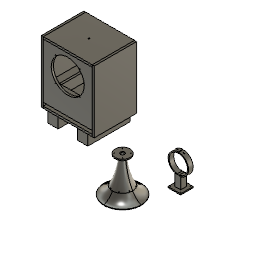
speaker-full-design (Autodesk Fusion 360 design; units mm, degrees)
Autodesk Fusion 360 part; units mm, degrees
sketch "HornProfile" plane through (0, 0, 0) normal (0, 1, 0) x (1, 0, 0)
  spline S0 degree 5 poles (18, 0) (18.0182, 0.1631) (18.0556, 0.496) (18.1141, 1.0154) (18.1973, 1.7477) (18.3097, 2.7291) (18.4304, 3.7743) (18.5588, 4.8793) (18.6943, 6.0374) (18.8359, 7.2396) (18.9826, 8.4763) (19.1333, 9.7379) (19.2872, 11.0163) (19.4438, 12.3059) (19.6027, 13.6042) (19.764, 14.9104) (19.9278, 16.2251) (20.0942, 17.5496) (20.2635, 18.8851) (20.4356, 20.2317) (20.6106, 21.5889) (20.7883, 22.9555) (20.9685, 24.3298) (21.1511, 25.7103) (21.3359, 27.0955) (21.5229, 28.4844) (21.7119, 29.8765) (21.903, 31.2715) (22.0963, 32.6694) (22.2917, 34.0701) (22.4893, 35.4739) (22.6891, 36.8805) (22.8911, 38.2897) (23.0954, 39.7013) (23.3018, 41.1147) (23.5104, 42.5296) (23.721, 43.9456) (23.9337, 45.3623) (24.1485, 46.7795) (24.3653, 48.1969) (24.5841, 49.6145) (24.8048, 51.0322) (25.0276, 52.4497) (25.2523, 53.8671) (25.4789, 55.2843) (25.7076, 56.701) (25.9382, 58.1171) (26.1709, 59.5326) (26.4056, 60.9472) (26.6423, 62.3607) (26.881, 63.7732) (27.1218, 65.1844) (27.3646, 66.5942) (27.6094, 68.0027) (27.8562, 69.4096) (28.1051, 70.8149) (28.3559, 72.2186) (28.6086, 73.6205) (28.8634, 75.0205) (29.12, 76.4187) (29.3787, 77.8149) (29.6393, 79.209) (29.9019, 80.6009) (30.1664, 81.9907) (30.4329, 83.3782) (30.7015, 84.7635) (30.972, 86.1463) (31.2446, 87.5268) (31.5193, 88.9048) (31.796, 90.2803) (32.0747, 91.6533) (32.3554, 93.0236) (32.6382, 94.3914) (32.923, 95.7564) (33.2098, 97.1188) (33.4986, 98.4784) (33.7894, 99.8352) (34.0822, 101.1892) (34.377, 102.5404) (34.6739, 103.8886) (34.9728, 105.234) (35.2737, 106.5763) (35.5767, 107.9157) (35.8817, 109.2521) (36.1887, 110.5855) (36.4978, 111.9158) (36.8089, 113.2431) (37.1221, 114.5672) (37.4374, 115.8882) (37.7548, 117.206) (38.0742, 118.5207) (38.3958, 119.8321) (38.7195, 121.1402) (39.0453, 122.4451) (39.3731, 123.7468) (39.703, 125.0451) (40.035, 126.3402) (40.3691, 127.6319) (40.7052, 128.9203) (41.0434, 130.2054) (41.3837, 131.4872) (41.7261, 132.7655) (42.0706, 134.0405) (42.4173, 135.312) (42.7661, 136.5802) (43.1172, 137.8448) (43.4704, 139.1061) (43.8258, 140.3639) (44.1834, 141.6182) (44.5432, 142.8691) (44.9051, 144.1166) (45.2692, 145.3605) (45.6354, 146.601) (46.0038, 147.8379) (46.3742, 149.0713) (46.7469, 150.3012) (47.1216, 151.5274) (47.4986, 152.7501) (47.8777, 153.9692) (48.259, 155.1847) (48.6425, 156.3966) (49.0283, 157.6049) (49.4163, 158.8096) (49.8065, 160.0107) (50.199, 161.2082) (50.5937, 162.4021) (50.9907, 163.5923) (51.3899, 164.779) (51.7913, 165.962) (52.195, 167.1413) (52.601, 168.317) (53.0092, 169.489) (53.4196, 170.6573) (53.8323, 171.8219) (54.2472, 172.9828) (54.6644, 174.14) (55.0838, 175.2935) (55.5055, 176.4433) (55.9295, 177.5894) (56.3557, 178.7317) (56.7843, 179.8702) (57.2153, 181.005) (57.6485, 182.136) (58.0842, 183.2632) (58.5222, 184.3866) (58.9625, 185.5062) (59.4051, 186.6222) (59.85, 187.7344) (60.2973, 188.8429) (60.7468, 189.9476) (61.1986, 191.0485) (61.6528, 192.1456) (62.1093, 193.2387) (62.5682, 194.328) (63.0294, 195.4134) (63.493, 196.4949) (63.959, 197.5725) (64.4274, 198.6463) (64.8982, 199.7163) (65.3713, 200.7825) (65.8469, 201.8448) (66.3248, 202.9033) (66.8051, 203.9579) (67.2879, 205.0085) (67.7731, 206.0552) (68.2607, 207.098) (68.7508, 208.1367) (69.2432, 209.1715) (69.7381, 210.2022) (70.2355, 211.229) (70.7353, 212.2518) (71.2375, 213.2707) (71.7422, 214.2855) (72.2493, 215.2964) (72.7589, 216.3032) (73.2711, 217.3061) (73.7857, 218.3049) (74.3028, 219.2997) (74.8225, 220.2904) (75.3446, 221.2771) (75.8692, 222.2597) (76.3962, 223.2382) (76.9256, 224.2126) (77.4575, 225.1829) (77.9918, 226.1491) (78.5286, 227.1111) (79.068, 228.0689) (79.6101, 229.0226) (80.1547, 229.9721) (80.702, 230.9174) (81.2518, 231.8585) (81.8041, 232.7954) (82.3589, 233.7281) (82.9162, 234.6566) (83.4759, 235.5808) (84.0382, 236.5007) (84.6031, 237.4163) (85.1705, 238.3276) (85.7407, 239.2346) (86.3134, 240.1371) (86.8888, 241.0353) (87.4668, 241.9291) (88.0473, 242.8185) (88.6305, 243.7035) (89.2162, 244.584) (89.8046, 245.46) (90.3956, 246.3316) (90.9893, 247.1987) (91.5856, 248.0613) (92.1845, 248.9195) (92.7861, 249.7731) (93.3903, 250.6223) (93.9971, 251.4669) (94.6066, 252.3068) (95.2187, 253.1421) (95.8334, 253.9726) (96.4508, 254.7984) (97.0709, 255.6194) (97.6936, 256.4356) (98.3191, 257.2471) (98.9473, 258.0539) (99.5782, 258.856) (100.2118, 259.6533) (100.8481, 260.4457) (101.4872, 261.2331) (102.1289, 262.0156) (102.7733, 262.7931) (103.4203, 263.5655) (104.07, 264.333) (104.7224, 265.0955) (105.3775, 265.853) (106.0354, 266.6053) (106.6961, 267.3526) (107.3596, 268.0946) (108.0259, 268.8313) (108.6951, 269.5628) (109.367, 270.289) (110.0416, 271.0098) (110.7189, 271.7253) (111.3989, 272.4355) (112.0817, 273.1401) (112.7674, 273.8392) (113.4559, 274.5328) (114.1473, 275.2207) (114.8415, 275.903) (115.5385, 276.5797) (116.2382, 277.2507) (116.9406, 277.916) (117.6458, 278.5755) (118.3539, 279.2291) (119.0648, 279.8767) (119.7786, 280.5183) (120.4953, 281.1537) (121.2148, 281.783) (121.9372, 282.4062) (122.6623, 283.0231) (123.3903, 283.6337) (124.1212, 284.2379) (124.855, 284.8357) (125.5918, 285.4269) (126.3316, 286.0114) (127.0742, 286.5893) (127.8197, 287.1603) (128.5679, 287.7245) (129.3189, 288.2817) (130.0727, 288.8319) (130.8295, 289.3751) (131.5893, 289.9111) (132.3522, 290.4399) (133.118, 290.9611) (133.8868, 291.4747) (134.6585, 291.9805) (135.4331, 292.4784) (136.2105, 292.9683) (136.9908, 293.4501) (137.7741, 293.9238) (138.5603, 294.3893) (139.3495, 294.8464) (140.1417, 295.2948) (140.9369, 295.7343) (141.7351, 296.1647) (142.5363, 296.5857) (143.3405, 296.9972) (144.1476, 297.3988) (144.9577, 297.7905) (145.7708, 298.1719) (146.587, 298.5428) (147.4062, 298.9029) (148.2284, 299.2517) (149.0536, 299.5887) (149.8818, 299.9134) (150.7129, 300.2253) (151.547, 300.5242) (152.3841, 300.8099) (153.2243, 301.082) (154.0677, 301.3397) (154.9142, 301.5811) (155.7639, 301.8038) (156.6167, 302.0054) (157.4725, 302.1836) (158.3314, 302.337) (159.0209, 302.4394) (159.5394, 302.5047) (159.8857, 302.5431) (160.059, 302.561) knots 0 0 0 0 0 0 0.00333333 0.00666667 0.01 0.01333333 0.01666667 0.02 0.02333333 0.02666667 0.03 0.03333333 0.03666667 0.04 0.04333333 0.04666667 0.05 0.05333333 0.05666667 0.06 0.06333333 0.06666667 0.07 0.07333333 0.07666667 0.08 0.08333333 0.08666667 0.09 0.09333333 0.09666667 0.1 0.10333333 0.10666667 0.11 0.11333333 0.11666667 0.12 0.12333333 0.12666667 0.13 0.13333333 0.13666667 0.14 0.14333333 0.14666667 0.15 0.15333333 0.15666667 0.16 0.16333333 0.16666667 0.17 0.17333333 0.17666667 0.18 0.18333333 0.18666667 0.19 0.19333333 0.19666667 0.2 0.20333333 0.20666667 0.21 0.21333333 0.21666667 0.22 0.22333333 0.22666667 0.23 0.23333333 0.23666667 0.24 0.24333333 0.24666667 0.25 0.25333333 0.25666667 0.26 0.26333333 0.26666667 0.27 0.27333333 0.27666667 0.28 0.28333333 0.28666667 0.29 0.29333333 0.29666667 0.3 0.30333333 0.30666667 0.31 0.31333333 0.31666667 0.32 0.32333333 0.32666667 0.33 0.33333333 0.33666667 0.34 0.34333333 0.34666667 0.35 0.35333333 0.35666667 0.36 0.36333333 0.36666667 0.37 0.37333333 0.37666667 0.38 0.38333333 0.38666667 0.39 0.39333333 0.39666667 0.4 0.40333333 0.40666667 0.41 0.41333333 0.41666667 0.42 0.42333333 0.42666667 0.43 0.43333333 0.43666667 0.44 0.44333333 0.44666667 0.45 0.45333333 0.45666667 0.46 0.46333333 0.46666667 0.47 0.47333333 0.47666667 0.48 0.48333333 0.48666667 0.49 0.49333333 0.49666667 0.5 0.50333333 0.50666667 0.51 0.51333333 0.51666667 0.52 0.52333333 0.52666667 0.53 0.53333333 0.53666667 0.54 0.54333333 0.54666667 0.55 0.55333333 0.55666667 0.56 0.56333333 0.56666667 0.57 0.57333333 0.57666667 0.58 0.58333333 0.58666667 0.59 0.59333333 0.59666667 0.6 0.60333333 0.60666667 0.61 0.61333333 0.61666667 0.62 0.62333333 0.62666667 0.63 0.63333333 0.63666667 0.64 0.64333333 0.64666667 0.65 0.65333333 0.65666667 0.66 0.66333333 0.66666667 0.67 0.67333333 0.67666667 0.68 0.68333333 0.68666667 0.69 0.69333333 0.69666667 0.7 0.70333333 0.70666667 0.71 0.71333333 0.71666667 0.72 0.72333333 0.72666667 0.73 0.73333333 0.73666667 0.74 0.74333333 0.74666667 0.75 0.75333333 0.75666667 0.76 0.76333333 0.76666667 0.77 0.77333333 0.77666667 0.78 0.78333333 0.78666667 0.79 0.79333333 0.79666667 0.8 0.80333333 0.80666667 0.81 0.81333333 0.81666667 0.82 0.82333333 0.82666667 0.83 0.83333333 0.83666667 0.84 0.84333333 0.84666667 0.85 0.85333333 0.85666667 0.86 0.86333333 0.86666667 0.87 0.87333333 0.87666667 0.88 0.88333333 0.88666667 0.89 0.89333333 0.89666667 0.9 0.90333333 0.90666667 0.91 0.91333333 0.91666667 0.92 0.92333333 0.92666667 0.93 0.93333333 0.93666667 0.94 0.94333333 0.94666667 0.95 0.95333333 0.95666667 0.96 0.96333333 0.96666667 0.97 0.97333333 0.97666667 0.98 0.98333333 0.98666667 0.99 0.99333333 0.99666667 1 1 1 1 1 1
  spline S1 degree 5 poles (23.961, -0.681) (23.9791, -0.5202) (24.016, -0.1922) (24.0738, 0.3193) (24.1559, 1.0402) (24.2665, 2.0055) (24.3851, 3.033) (24.5111, 4.1191) (24.6441, 5.2572) (24.783, 6.4388) (24.9269, 7.6547) (25.0748, 8.8956) (25.2261, 10.1535) (25.3799, 11.4227) (25.5362, 12.7005) (25.6948, 13.986) (25.8559, 15.2796) (26.0194, 16.5826) (26.1857, 17.8961) (26.3548, 19.2205) (26.5266, 20.5553) (26.7011, 21.8994) (26.878, 23.2514) (27.0574, 24.6097) (27.239, 25.9729) (27.4227, 27.3398) (27.6085, 28.7098) (27.7963, 30.0826) (27.9862, 31.4583) (28.1782, 32.8367) (28.3723, 34.218) (28.5685, 35.6021) (28.7669, 36.9889) (28.9672, 38.378) (29.1697, 39.7691) (29.3742, 41.1617) (29.5807, 42.5554) (29.7891, 43.9499) (29.9996, 45.3448) (30.212, 46.74) (30.4263, 48.1354) (30.6427, 49.5309) (30.861, 50.9263) (31.0814, 52.3215) (31.3037, 53.7166) (31.528, 55.1113) (31.7542, 56.5054) (31.9825, 57.8989) (32.2126, 59.2915) (32.4448, 60.6832) (32.6788, 62.0737) (32.9148, 63.463) (33.1527, 64.851) (33.3925, 66.2376) (33.6342, 67.6228) (33.8778, 69.0064) (34.1234, 70.3884) (34.3708, 71.7688) (34.6203, 73.1473) (34.8717, 74.524) (35.125, 75.8987) (35.3803, 77.2714) (35.6376, 78.642) (35.8969, 80.0104) (36.158, 81.3766) (36.4211, 82.7406) (36.6861, 84.1022) (36.953, 85.4615) (37.2218, 86.8185) (37.4925, 88.173) (37.7651, 89.5251) (38.0396, 90.8746) (38.316, 92.2216) (38.5945, 93.566) (38.8749, 94.9077) (39.1574, 96.2466) (39.4419, 97.5828) (39.7284, 98.9162) (40.0169, 100.2467) (40.3074, 101.5744) (40.5998, 102.8991) (40.8942, 104.221) (41.1906, 105.5399) (41.4889, 106.8558) (41.7892, 108.1688) (42.0914, 109.4788) (42.3957, 110.7858) (42.7019, 112.0897) (43.0101, 113.3906) (43.3203, 114.6884) (43.6325, 115.9831) (43.9466, 117.2746) (44.2627, 118.5628) (44.5808, 119.8479) (44.9008, 121.1297) (45.223, 122.4083) (45.5472, 123.6836) (45.8735, 124.9557) (46.202, 126.2245) (46.5325, 127.49) (46.8652, 128.7522) (47.1999, 130.0111) (47.5366, 131.2666) (47.8754, 132.5188) (48.2161, 133.7676) (48.5588, 135.0129) (48.9035, 136.2548) (49.2502, 137.4933) (49.599, 138.7284) (49.9499, 139.9601) (50.3029, 141.1883) (50.6581, 142.4131) (51.0155, 143.6344) (51.375, 144.8522) (51.7365, 146.0666) (52.1002, 147.2775) (52.4659, 148.4848) (52.8337, 149.6887) (53.2036, 150.8889) (53.5756, 152.0857) (53.9497, 153.2789) (54.326, 154.4685) (54.7044, 155.6545) (55.0849, 156.837) (55.4676, 158.016) (55.8524, 159.1913) (56.2394, 160.3631) (56.6284, 161.5313) (57.0195, 162.6959) (57.4128, 163.8569) (57.8082, 165.0143) (58.2058, 166.168) (58.6057, 167.318) (59.0077, 168.4644) (59.4119, 169.607) (59.8184, 170.746) (60.2271, 171.8813) (60.638, 173.0129) (61.0511, 174.1409) (61.4664, 175.2651) (61.8839, 176.3857) (62.3037, 177.5025) (62.7257, 178.6156) (63.15, 179.725) (63.5765, 180.8307) (64.0052, 181.9326) (64.4361, 183.0307) (64.8691, 184.1252) (65.3043, 185.2158) (65.7416, 186.3028) (66.1811, 187.3859) (66.623, 188.4653) (67.0671, 189.5408) (67.5136, 190.6125) (67.9625, 191.6804) (68.4137, 192.7444) (68.8673, 193.8046) (69.3232, 194.8609) (69.7813, 195.9135) (70.2416, 196.9622) (70.7041, 198.0071) (71.1687, 199.0483) (71.6357, 200.0855) (72.1049, 201.1189) (72.5765, 202.1484) (73.0504, 203.174) (73.5268, 204.1957) (74.0055, 205.2134) (74.4866, 206.2271) (74.97, 207.2369) (75.4558, 208.2427) (75.9439, 209.2446) (76.4344, 210.2425) (76.9271, 211.2364) (77.4222, 212.2264) (77.9196, 213.2125) (78.4192, 214.1945) (78.9212, 215.1727) (79.4256, 216.1468) (79.9323, 217.1168) (80.4414, 218.0828) (80.9529, 219.0447) (81.4668, 220.0025) (81.9832, 220.9561) (82.502, 221.9056) (83.0233, 222.851) (83.547, 223.7923) (84.0731, 224.7295) (84.6015, 225.6626) (85.1322, 226.5916) (85.6653, 227.5164) (86.2008, 228.4371) (86.7388, 229.3535) (87.2793, 230.2657) (87.8223, 231.1736) (88.3678, 232.0772) (88.9159, 232.9764) (89.4663, 233.8714) (90.0192, 234.7622) (90.5744, 235.6487) (91.132, 236.531) (91.6919, 237.409) (92.2542, 238.2826) (92.8189, 239.1518) (93.3861, 240.0167) (93.9559, 240.877) (94.5282, 241.7329) (95.103, 242.5843) (95.6805, 243.4311) (96.2605, 244.2735) (96.843, 245.1113) (97.428, 245.9447) (98.0153, 246.7735) (98.605, 247.5979) (99.1972, 248.4177) (99.7918, 249.2329) (100.389, 250.0434) (100.9888, 250.8493) (101.5912, 251.6503) (102.1961, 252.4467) (102.8036, 253.2382) (103.4135, 254.0248) (104.026, 254.8067) (104.6409, 255.5837) (105.2584, 256.3559) (105.8783, 257.1233) (106.5008, 257.8859) (107.1258, 258.6435) (107.7534, 259.3962) (108.3835, 260.144) (109.0162, 260.8866) (109.6513, 261.6241) (110.2891, 262.3565) (110.9294, 263.0838) (111.5723, 263.8058) (112.2178, 264.5226) (112.8659, 265.2341) (113.5166, 265.9404) (114.1698, 266.6414) (114.8255, 267.337) (115.4838, 268.0272) (116.1446, 268.712) (116.8079, 269.3912) (117.4739, 270.0649) (118.1425, 270.7329) (118.8137, 271.3953) (119.4874, 272.0521) (120.1636, 272.7032) (120.8424, 273.3486) (121.5236, 273.9882) (122.2074, 274.6218) (122.8938, 275.2495) (123.5828, 275.8711) (124.2744, 276.4866) (124.9686, 277.096) (125.6653, 277.6991) (126.3646, 278.296) (127.0664, 278.8866) (127.7707, 279.4707) (128.4775, 280.0484) (129.1869, 280.6195) (129.8989, 281.1839) (130.6134, 281.7416) (131.3304, 282.2925) (132.0499, 282.8366) (132.772, 283.3738) (133.4966, 283.9039) (134.2238, 284.4267) (134.9534, 284.942) (135.6856, 285.4499) (136.4202, 285.9502) (137.1571, 286.443) (137.8963, 286.9282) (138.6378, 287.4057) (139.3817, 287.8752) (140.1281, 288.3365) (140.877, 288.7894) (141.6283, 289.2336) (142.3818, 289.6691) (143.1375, 290.0958) (143.8951, 290.5134) (144.6548, 290.9219) (145.4168, 291.3209) (146.1812, 291.7101) (146.948, 292.0892) (147.7168, 292.458) (148.487, 292.8162) (149.2581, 293.1636) (150.03, 293.4998) (150.8036, 293.8244) (151.5798, 294.1369) (152.3591, 294.4366) (153.1407, 294.723) (153.9218, 294.9956) (154.6993, 295.2535) (155.4713, 295.4961) (156.2386, 295.722) (157.0056, 295.9295) (157.778, 296.1169) (158.5615, 296.2827) (159.36, 296.4258) (160.0121, 296.5219) (160.509, 296.5835) (160.8438, 296.62) (161.012, 296.637) knots 0 0 0 0 0 0 0.00333333 0.00666667 0.01 0.01333333 0.01666667 0.02 0.02333333 0.02666667 0.03 0.03333333 0.03666667 0.04 0.04333333 0.04666667 0.05 0.05333333 0.05666667 0.06 0.06333333 0.06666667 0.07 0.07333333 0.07666667 0.08 0.08333333 0.08666667 0.09 0.09333333 0.09666667 0.1 0.10333333 0.10666667 0.11 0.11333333 0.11666667 0.12 0.12333333 0.12666667 0.13 0.13333333 0.13666667 0.14 0.14333333 0.14666667 0.15 0.15333333 0.15666667 0.16 0.16333333 0.16666667 0.17 0.17333333 0.17666667 0.18 0.18333333 0.18666667 0.19 0.19333333 0.19666667 0.2 0.20333333 0.20666667 0.21 0.21333333 0.21666667 0.22 0.22333333 0.22666667 0.23 0.23333333 0.23666667 0.24 0.24333333 0.24666667 0.25 0.25333333 0.25666667 0.26 0.26333333 0.26666667 0.27 0.27333333 0.27666667 0.28 0.28333333 0.28666667 0.29 0.29333333 0.29666667 0.3 0.30333333 0.30666667 0.31 0.31333333 0.31666667 0.32 0.32333333 0.32666667 0.33 0.33333333 0.33666667 0.34 0.34333333 0.34666667 0.35 0.35333333 0.35666667 0.36 0.36333333 0.36666667 0.37 0.37333333 0.37666667 0.38 0.38333333 0.38666667 0.39 0.39333333 0.39666667 0.4 0.40333333 0.40666667 0.41 0.41333333 0.41666667 0.42 0.42333333 0.42666667 0.43 0.43333333 0.43666667 0.44 0.44333333 0.44666667 0.45 0.45333333 0.45666667 0.46 0.46333333 0.46666667 0.47 0.47333333 0.47666667 0.48 0.48333333 0.48666667 0.49 0.49333333 0.49666667 0.5 0.50333333 0.50666667 0.51 0.51333333 0.51666667 0.52 0.52333333 0.52666667 0.53 0.53333333 0.53666667 0.54 0.54333333 0.54666667 0.55 0.55333333 0.55666667 0.56 0.56333333 0.56666667 0.57 0.57333333 0.57666667 0.58 0.58333333 0.58666667 0.59 0.59333333 0.59666667 0.6 0.60333333 0.60666667 0.61 0.61333333 0.61666667 0.62 0.62333333 0.62666667 0.63 0.63333333 0.63666667 0.64 0.64333333 0.64666667 0.65 0.65333333 0.65666667 0.66 0.66333333 0.66666667 0.67 0.67333333 0.67666667 0.68 0.68333333 0.68666667 0.69 0.69333333 0.69666667 0.7 0.70333333 0.70666667 0.71 0.71333333 0.71666667 0.72 0.72333333 0.72666667 0.73 0.73333333 0.73666667 0.74 0.74333333 0.74666667 0.75 0.75333333 0.75666667 0.76 0.76333333 0.76666667 0.77 0.77333333 0.77666667 0.78 0.78333333 0.78666667 0.79 0.79333333 0.79666667 0.8 0.80333333 0.80666667 0.81 0.81333333 0.81666667 0.82 0.82333333 0.82666667 0.83 0.83333333 0.83666667 0.84 0.84333333 0.84666667 0.85 0.85333333 0.85666667 0.86 0.86333333 0.86666667 0.87 0.87333333 0.87666667 0.88 0.88333333 0.88666667 0.89 0.89333333 0.89666667 0.9 0.90333333 0.90666667 0.91 0.91333333 0.91666667 0.92 0.92333333 0.92666667 0.93 0.93333333 0.93666667 0.94 0.94333333 0.94666667 0.95 0.95333333 0.95666667 0.96 0.96333333 0.96666667 0.97 0.97333333 0.97666667 0.98 0.98333333 0.98666667 0.99 0.99333333 0.99666667 1 1 1 1 1 1
  line L0 (18, 0) -> (23.961, -0.681)
  line L1 (160.059, 302.561) -> (161.012, 296.637)
  point P0 (18.46, 4.028)
  point P1 (19.215, 10.415)
  point P2 (20.143, 17.933)
  point P3 (21.206, 26.12)
  point P4 (22.381, 34.703)
  point P5 (23.655, 43.5)
  point P6 (25.018, 52.386)
  point P7 (26.46, 61.27)
  point P8 (27.977, 70.09)
  point P9 (29.563, 78.799)
  point P10 (31.213, 87.364)
  point P11 (32.925, 95.763)
  point P12 (34.695, 103.981)
  point P13 (36.52, 112.008)
  point P14 (38.398, 119.838)
  point P15 (40.327, 127.467)
  point P16 (42.304, 134.895)
  point P17 (44.329, 142.123)
  point P18 (46.4, 149.154)
  point P19 (48.514, 155.989)
  point P20 (50.671, 162.632)
  point P21 (52.87, 169.088)
  point P22 (55.109, 175.36)
  point P23 (57.387, 181.452)
  point P24 (59.704, 187.368)
  point P25 (62.058, 193.114)
  point P26 (64.448, 198.691)
  point P27 (66.874, 204.106)
  point P28 (69.335, 209.361)
  point P29 (71.83, 214.459)
  point P30 (74.359, 219.405)
  point P31 (76.921, 224.202)
  point P32 (79.514, 228.852)
  point P33 (82.14, 233.359)
  point P34 (84.796, 237.725)
  point P35 (87.483, 241.952)
  point P36 (90.2, 246.042)
  point P37 (92.947, 249.998)
  point P38 (95.723, 253.822)
  point P39 (98.527, 257.513)
  point P40 (101.36, 261.075)
  point P41 (104.22, 264.507)
  point P42 (107.107, 267.811)
  point P43 (110.022, 270.987)
  point P44 (112.963, 274.035)
  point P45 (115.931, 276.955)
  point P46 (118.924, 279.747)
  point P47 (121.943, 282.409)
  point P48 (124.987, 284.94)
  point P49 (128.057, 287.338)
  point P50 (131.15, 289.6)
  point P51 (134.269, 291.724)
  point P52 (137.411, 293.703)
  point P53 (140.577, 295.534)
  point P54 (143.767, 297.208)
  point P55 (146.98, 298.714)
  point P56 (150.216, 300.037)
  point P57 (153.474, 301.156)
  point P58 (156.756, 302.03)
  point P59 (24.42, 3.333)
  point P60 (25.171, 9.694)
  point P61 (26.095, 17.178)
  point P62 (27.153, 25.326)
  point P63 (28.323, 33.865)
  point P64 (29.59, 42.615)
  point P65 (30.944, 51.45)
  point P66 (32.378, 60.281)
  point P67 (33.885, 69.044)
  point P68 (35.46, 77.694)
  point P69 (37.099, 86.197)
  point P70 (38.797, 94.533)
  point P71 (40.553, 102.685)
  point P72 (42.363, 110.643)
  point P73 (44.224, 118.403)
  point P74 (46.134, 125.96)
  point P75 (48.093, 133.315)
  point P76 (50.096, 140.467)
  point P77 (52.144, 147.42)
  point P78 (54.234, 154.176)
  point P79 (56.365, 160.739)
  point P80 (58.535, 167.113)
  point P81 (60.744, 173.301)
  point P82 (62.991, 179.308)
  point P83 (65.274, 185.138)
  point P84 (67.591, 190.795)
  point P85 (69.944, 196.283)
  point P86 (72.329, 201.607)
  point P87 (74.747, 206.77)
  point P88 (77.197, 211.775)
  point P89 (79.677, 216.627)
  point P90 (82.187, 221.328)
  point P91 (84.727, 225.881)
  point P92 (87.295, 230.29)
  point P93 (89.892, 234.556)
  point P94 (92.515, 238.683)
  point P95 (95.164, 242.672)
  point P96 (97.84, 246.525)
  point P97 (100.54, 250.245)
  point P98 (103.265, 253.832)
  point P99 (106.013, 257.287)
  point P100 (108.784, 260.613)
  point P101 (111.577, 263.809)
  point P102 (114.392, 266.876)
  point P103 (117.227, 269.814)
  point P104 (120.082, 272.623)
  point P105 (122.955, 275.303)
  point P106 (125.846, 277.852)
  point P107 (128.753, 280.269)
  point P108 (131.675, 282.552)
  point P109 (134.611, 284.699)
  point P110 (137.558, 286.705)
  point P111 (140.513, 288.568)
  point P112 (143.474, 290.28)
  point P113 (146.435, 291.834)
  point P114 (149.39, 293.219)
  point P115 (152.327, 294.421)
  point P116 (155.223, 295.416)
  point P117 (158.008, 296.162)
revolve "Revolve1" add sketch "HornProfile" angle 360 about axis through (0, 0, 1.75) along (0, 0, 1) makes body 1
sketch "Flange" plane through (0, 0, 0) normal (0, 0, 1) x (1, 0, 0)
  circle A0 centre (0, 0) radius 18
  circle A1 centre (0, 0) radius 65
extrude "Extrude1" add sketch "Flange" along normal blind 8 and the other way blind 2 bodies 1
sketch "FlangeBolts" plane through (0, 0, 0) normal (0, 0, 1) x (1, 0, 0)
  circle A0 centre (36.0624, 36.0624) radius 3.25
  circle A1 centre (-36.0624, 36.0624) radius 3.25
  circle A2 centre (-36.0624, -36.0624) radius 3.25
  circle A3 centre (36.0624, -36.0624) radius 3.25
extrude "Extrude2" cut sketch "FlangeBolts" along normal blind 10 and the other way blind 4 bodies 1
ref_plane "WorkPlane1" through (0, 0, -230) normal (0, 0, 1) x (1, 0, 0)
sketch "RingPins" plane through (0, 0, -230) normal (0, 0, 1) x (1, 0, 0)
  circle A0 centre (72.3131, 41.75) radius 2
  circle A1 centre (21.6114, 80.6548) radius 2
  circle A2 centre (-41.75, 72.3131) radius 2
  circle A3 centre (-80.6548, 21.6114) radius 2
  circle A4 centre (-72.3131, -41.75) radius 2
  circle A5 centre (-21.6114, -80.6548) radius 2
  circle A6 centre (41.75, -72.3131) radius 2
  circle A7 centre (80.6548, -21.6114) radius 2
extrude "Extrude3" cut sketch "RingPins" along normal blind 10 and the other way blind 10 bodies 1
split "Split1" by plane through (0, 0, -230) normal (0, 0, 1) bodies 1 makes body 2 at (69.6941, -25.494, -205.6445)
split "Split2" by plane through (0, 0, 0) normal (0, 1, 0) bodies 1 makes body 3 at (89.0358, 54.3131, -264.5939)
split "Split3" by plane through (0, 0, 0) normal (1, 0, 0) bodies 1 makes body 4 at (65.2917, -81.1234, -264.4068)
split "Split4" by plane through (0, 0, 0) normal (1, 0, 0) bodies 3 makes body 5 at (75.5013, 71.5991, -264.3101)
sketch "StandBase" plane through (0, 0, 0) normal (0, 0, 1) x (1, 0, 0)
  line L0 (455, -45) -> (545, -45)
  line L1 (545, -45) -> (545, 45)
  line L2 (545, 45) -> (455, 45)
  line L3 (455, 45) -> (455, -45)
extrude "Extrude4" add sketch "StandBase" along normal blind 8 and the other way blind 0 separate body makes body 6
sketch "StandCol" plane through (0, 0, 0) normal (0, 0, 1) x (1, 0, 0)
  line L0 (480, -20) -> (520, -20)
  line L1 (520, -20) -> (520, 20)
  line L2 (520, 20) -> (480, 20)
  line L3 (480, 20) -> (480, -20)
extrude "Extrude5" add sketch "StandCol" along normal blind 113 bodies 6
sketch "StandRing" plane through (0, 0, 0) normal (0, 1, 0) x (1, 0, 0)
  circle A0 centre (500, -188) radius 63
  circle A1 centre (500, -188) radius 75
extrude "Extrude6" add sketch "StandRing" along normal blind 20 and the other way blind 20 bodies 6
sketch "StandSlot" plane through (0, 0, 0) normal (0, 0, 1) x (1, 0, 0)
  line L0 (498, -21) -> (502, -21)
  line L1 (502, -21) -> (502, 21)
  line L2 (502, 21) -> (498, 21)
  line L3 (498, 21) -> (498, -21)
extrude "Extrude7" cut sketch "StandSlot" along normal blind 270 and the other way blind -188 bodies 6
sketch "ClampBolt" plane through (0, 0, 0) normal (1, 0, 0) x (0, 0, -1)
  circle A0 centre (-257, 0) radius 2.6
extrude "Extrude8" cut sketch "ClampBolt" along normal blind 535 and the other way blind 535 bodies 6
sketch "BaseScrews" plane through (0, 0, 0) normal (0, 0, 1) x (1, 0, 0)
  circle A0 centre (465, -35) radius 2.25
  circle A1 centre (465, 35) radius 2.25
  circle A2 centre (535, -35) radius 2.25
  circle A3 centre (535, 35) radius 2.25
extrude "Extrude9" cut sketch "BaseScrews" along normal blind 10 and the other way blind 1 bodies 6
ref_plane "WorkPlane2" through (0, 0, 0) normal (0, 0, 1) x (1, 0, 0)
sketch "sk_Cab_SideL" plane through (0, 0, 0) normal (0, 0, 1) x (1, 0, 0)
  line L0 (-700, 0) -> (-682, 0)
  line L1 (-682, 0) -> (-682, 366)
  line L2 (-682, 366) -> (-700, 366)
  line L3 (-700, 366) -> (-700, 0)
extrude "Extrude10" add sketch "sk_Cab_SideL" along normal blind 536 separate body makes body 7
ref_plane "WorkPlane3" through (0, 0, 0) normal (0, 0, 1) x (1, 0, 0)
sketch "sk_Cab_SideR" plane through (0, 0, 0) normal (0, 0, 1) x (1, 0, 0)
  line L0 (-262, 0) -> (-244, 0)
  line L1 (-244, 0) -> (-244, 366)
  line L2 (-244, 366) -> (-262, 366)
  line L3 (-262, 366) -> (-262, 0)
extrude "Extrude11" add sketch "sk_Cab_SideR" along normal blind 536 separate body makes body 8
ref_plane "WorkPlane4" through (0, 0, 0) normal (0, 0, 1) x (1, 0, 0)
sketch "sk_Cab_Bottom" plane through (0, 0, 0) normal (0, 0, 1) x (1, 0, 0)
  line L0 (-682, 0) -> (-262, 0)
  line L1 (-262, 0) -> (-262, 366)
  line L2 (-262, 366) -> (-682, 366)
  line L3 (-682, 366) -> (-682, 0)
extrude "Extrude12" add sketch "sk_Cab_Bottom" along normal blind 18 separate body makes body 9
ref_plane "WorkPlane5" through (0, 0, 518) normal (0, 0, 1) x (1, 0, 0)
sketch "sk_Cab_Top" plane through (0, 0, 518) normal (0, 0, 1) x (1, 0, 0)
  line L0 (-682, 0) -> (-262, 0)
  line L1 (-262, 0) -> (-262, 366)
  line L2 (-262, 366) -> (-682, 366)
  line L3 (-682, 366) -> (-682, 0)
extrude "Extrude13" add sketch "sk_Cab_Top" along normal blind 18 separate body makes body 10
ref_plane "WorkPlane6" through (0, 0, 18) normal (0, 0, 1) x (1, 0, 0)
sketch "sk_Cab_Back" plane through (0, 0, 18) normal (0, 0, 1) x (1, 0, 0)
  line L0 (-682, 348) -> (-262, 348)
  line L1 (-262, 348) -> (-262, 366)
  line L2 (-262, 366) -> (-682, 366)
  line L3 (-682, 366) -> (-682, 348)
extrude "Extrude14" add sketch "sk_Cab_Back" along normal blind 500 separate body makes body 11
ref_plane "WorkPlane7" through (0, 0, 46) normal (0, 0, 1) x (1, 0, 0)
sketch "sk_Cab_Baffle" plane through (0, 0, 46) normal (0, 0, 1) x (1, 0, 0)
  line L0 (-682, 0) -> (-262, 0)
  line L1 (-262, 0) -> (-262, 18)
  line L2 (-262, 18) -> (-682, 18)
  line L3 (-682, 18) -> (-682, 0)
extrude "Extrude15" add sketch "sk_Cab_Baffle" along normal blind 472 separate body makes body 12
ref_plane "WorkPlane8" through (0, 0, 46) normal (0, 0, 1) x (1, 0, 0)
sketch "sk_Cab_PortShelf" plane through (0, 0, 46) normal (0, 0, 1) x (1, 0, 0)
  line L0 (-682, 0) -> (-262, 0)
  line L1 (-262, 0) -> (-262, 150)
  line L2 (-262, 150) -> (-682, 150)
  line L3 (-682, 150) -> (-682, 0)
extrude "Extrude16" add sketch "sk_Cab_PortShelf" along normal blind 18 separate body makes body 13
ref_plane "WorkPlane9" through (0, 0, 160) normal (0, 0, 1) x (1, 0, 0)
sketch "sk_Cab_Brace" plane through (0, 0, 160) normal (0, 0, 1) x (1, 0, 0)
  line L0 (-682, 18) -> (-262, 18)
  line L1 (-262, 18) -> (-262, 348)
  line L2 (-262, 348) -> (-682, 348)
  line L3 (-682, 348) -> (-682, 18)
extrude "Extrude17" add sketch "sk_Cab_Brace" along normal blind 18 separate body makes body 14
ref_plane "WorkPlane10" through (0, 0, -90) normal (0, 0, 1) x (1, 0, 0)
sketch "sk_Cab_FootL" plane through (0, 0, -90) normal (0, 0, 1) x (1, 0, 0)
  line L0 (-645, 0) -> (-555, 0)
  line L1 (-555, 0) -> (-555, 366)
  line L2 (-555, 366) -> (-645, 366)
  line L3 (-645, 366) -> (-645, 0)
extrude "Extrude18" add sketch "sk_Cab_FootL" along normal blind 90 separate body makes body 15
ref_plane "WorkPlane11" through (0, 0, -90) normal (0, 0, 1) x (1, 0, 0)
sketch "sk_Cab_FootR" plane through (0, 0, -90) normal (0, 0, 1) x (1, 0, 0)
  line L0 (-389, 0) -> (-299, 0)
  line L1 (-299, 0) -> (-299, 366)
  line L2 (-299, 366) -> (-389, 366)
  line L3 (-389, 366) -> (-389, 0)
extrude "Extrude19" add sketch "sk_Cab_FootR" along normal blind 90 separate body makes body 16
sketch "WooferCut" plane through (0, 0, 0) normal (0, 1, 0) x (1, 0, 0)
  circle A0 centre (-472, -346) radius 141.5
  circle A1 centre (-366.9946, -451.0054) radius 3.5
  circle A2 centre (-577.0054, -451.0054) radius 3.5
  circle A3 centre (-577.0054, -240.9946) radius 3.5
  circle A4 centre (-366.9946, -240.9946) radius 3.5
extrude "Extrude20" cut sketch "WooferCut" along normal blind 400 and the other way blind 400 bodies 12
sketch "TerminalCut" plane through (0, 0, 0) normal (0, 1, 0) x (1, 0, 0)
  circle A0 centre (-472, -100) radius 30
extrude "Extrude21" cut sketch "TerminalCut" along normal blind 400 and the other way blind 400 bodies 11
sketch "BraceWindow" plane through (0, 0, 0) normal (0, 0, 1) x (1, 0, 0)
  line L0 (-622, 78) -> (-322, 78)
  line L1 (-322, 78) -> (-322, 288)
  line L2 (-322, 288) -> (-622, 288)
  line L3 (-622, 288) -> (-622, 78)
extrude "Extrude22" cut sketch "BraceWindow" along normal blind 200 and the other way blind 10 bodies 14
sketch "CableExit" plane through (0, 0, 0) normal (0, 0, 1) x (1, 0, 0)
  circle A0 centre (-472, 183) radius 5
extrude "Extrude23" cut sketch "CableExit" along normal blind 540 and the other way blind 10 bodies 10
ref_plane "WorkPlane12" through (0, 0, 18) normal (0, 0, 1) x (1, 0, 0)
sketch "AirBox" plane through (0, 0, 18) normal (0, 0, 1) x (1, 0, 0)
  line L0 (-682, 18) -> (-262, 18)
  line L1 (-262, 18) -> (-262, 348)
  line L2 (-262, 348) -> (-682, 348)
  line L3 (-682, 348) -> (-682, 18)
extrude "Extrude24" add sketch "AirBox" along normal blind 500 separate body makes body 17
combine "Combine1" operation cut target body 17 tool bodies 13 keep tools
combine "Combine2" operation cut target body 17 tool bodies 14 keep tools
sketch "DuctCut" plane through (0, 0, 18) normal (0, 0, 1) x (1, 0, 0)
  line L0 (-682, 18) -> (-262, 18)
  line L1 (-262, 18) -> (-262, 150)
  line L2 (-262, 150) -> (-682, 150)
  line L3 (-682, 150) -> (-682, 18)
extrude "Extrude25" cut sketch "DuctCut" along normal blind 28 bodies 17
combine "Combine3" operation cut target body 13 tool bodies 12 keep tools
delete_body "RemoveBody1" bodies 17
delete_body "RemoveBody2" bodies 6
sketch "StandBase2" plane through (0, 0, 0) normal (0, 0, 1) x (1, 0, 0)
  line L0 (445, -55) -> (555, -55)
  line L1 (555, -55) -> (555, 55)
  line L2 (555, 55) -> (445, 55)
  line L3 (445, 55) -> (445, -55)
extrude "Extrude26" add sketch "StandBase2" along normal blind 10 separate body makes body 18
sketch "StandCol2" plane through (0, 0, 0) normal (0, 0, 1) x (1, 0, 0)
  line L0 (475, -25) -> (525, -25)
  line L1 (525, -25) -> (525, 25)
  line L2 (525, 25) -> (475, 25)
  line L3 (475, 25) -> (475, -25)
extrude "Extrude27" add sketch "StandCol2" along normal blind 110 bodies 18
sketch "StandRing2" plane through (0, 0, 0) normal (0, 1, 0) x (1, 0, 0)
  circle A0 centre (500, -188) radius 78.5
  circle A1 centre (500, -188) radius 88.5
extrude "Extrude28" add sketch "StandRing2" along normal blind 20 and the other way blind 20 bodies 18
ref_plane "WorkPlane13" through (0, 0, 188) normal (0, 0, 1) x (1, 0, 0)
sketch "StandSlot2" plane through (0, 0, 188) normal (0, 0, 1) x (1, 0, 0)
  line L0 (498, -21) -> (502, -21)
  line L1 (502, -21) -> (502, 21)
  line L2 (502, 21) -> (498, 21)
  line L3 (498, 21) -> (498, -21)
extrude "Extrude29" cut sketch "StandSlot2" along normal blind 105 bodies 18
sketch "ClampBolt2" plane through (0, 0, 0) normal (1, 0, 0) x (0, 0, -1)
  circle A0 centre (-272, 0) radius 2.6
extrude "Extrude30" cut sketch "ClampBolt2" along normal blind 535 and the other way blind 535 bodies 18
sketch "BaseScrews2" plane through (0, 0, 0) normal (0, 0, 1) x (1, 0, 0)
  circle A0 centre (457, -43) radius 2.25
  circle A1 centre (457, 43) radius 2.25
  circle A2 centre (543, -43) radius 2.25
  circle A3 centre (543, 43) radius 2.25
extrude "Extrude31" cut sketch "BaseScrews2" along normal blind 12 and the other way blind 1 bodies 18
named bodies: "Horn_Bell_Q1", "Horn_Neck", "Horn_Bell_Q2", "Horn_Bell_Q3", "Horn_Bell_Q4", "DriverStand", "Cab_SideL", "Cab_SideR", "Cab_Bottom", "Cab_Top", "Cab_Back", "Cab_Baffle", "Cab_PortShelf", "Cab_Brace", "Cab_FootL", "Cab_FootR", "AirCheck"
